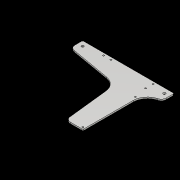
# Autodesk Inventor part: small_gpu_04
Saved by Autodesk Inventor 2018.2 (Build 222227000, 227)
## iProperties
Created: 2020-06-13
Part Number: small_gpu_04
Material: アルミニウム 6061
Document SubType Name: Modeling
Designer: gisen
Density: 2.7 g/cm^3
Appearance: アルミニウム - フラット
Author: gisen
Autodesk Inventor part; units mm, degrees
ref_plane "YZ Plane" through (0, 0, 0) normal (1, 0, 0) x (0, 1, 0)
ref_plane "XZ Plane" through (0, 0, 0) normal (0, 1, 0) x (-1, 0, 0)
ref_plane "XY Plane" through (0, 0, 0) normal (0, 0, 1) x (1, 0, 0)
sketch "スケッチ1" plane through (0, 0, 0) normal (0, 0, 1) x (1, 0, 0)
  line L0 (0, 0) -> (130.16, 0)
  line L1 (130.16, 0) -> (130.16, 159.597)
  line L2 (130.16, 159.597) -> (0, 159.597)
  line L3 (0, 159.597) -> (0, 0)
  dimension "d0" = 130.16
  dimension "d1" = 159.597
  constraints: 8 end point, 2 parallel, 1 horizontal, 1 perpendicular
  measures "d0" distance of L1.end L2.end
  measures "d1" distance between parallel lines of L0 L2
extrude "押し出し1" add sketch "スケッチ1" along normal blind 3
sketch "スケッチ2" plane through (0, 0, 3) normal (0, 0, 1) x (1, 0, 0)
  line L0 (126.16, 3.92) -> (126.16, 113.08) construction
  circle A0 centre (126.16, 3.92) radius 1.6
  circle A1 centre (126.16, 113.08) radius 1.6
  line L1 (130.16, 0) -> (130.16, 159.597) projected
  line L2 (0, 0) -> (130.16, 0) projected
  circle A2 centre (121.531, 154.597) radius 1.6
  line L3 (130.16, 159.597) -> (0, 159.597) projected
  line L4 (121.531, 154.597) -> (121.531, 139.097) construction
  circle A3 centre (121.531, 139.097) radius 1.6
  line L5 (18.398, 154.597) -> (33.898, 154.597) construction
  line L6 (0, 159.597) -> (0, 0) construction
  circle A4 centre (18.398, 154.597) radius 1.6
  circle A5 centre (33.898, 154.597) radius 1.6
  dimension "d4" = 3.2
  dimension "d5" = 4
  dimension "d6" = 3.92
  dimension "d7" = 109.16
  dimension "d10" = 5
  dimension "d11" = 8.629
  dimension "d12" = 15.5
  dimension "d13" = 18.398
  dimension "d14" = 5
  dimension "d15" = 15.5
  constraints: 6 centre point, 6 end point, 5 coincident, 5 equal radius, 2 vertical, 1 horizontal
  measures "d4" diameter of A0
  measures "d5" distance between parallel lines of L1 L0
  measures "d6" distance from line of L2 L0.start
  measures "d7" distance of L0.start L0.end
  measures "d10" distance from line of L4.start L3
  measures "d11" distance from line of L1 L4.start
  measures "d12" distance of L4.start L4.end
  measures "d13" distance from line of L6 L5.start
  measures "d14" distance between parallel lines of L5 L3
  measures "d15" distance of L5.start L5.end
extrude "押し出し2" cut sketch "スケッチ2" against normal blind 3
sketch "スケッチ4" plane through (0, 0, 3) normal (0, 0, 1) x (1, 0, 0)
  line L0 (130.16, 159.597) -> (0, 159.597) construction
  line L1 (130.16, 0) -> (130.16, 159.597) construction
  line L2 (0, 159.597) -> (0, 0) construction
  line L3 (0, 159.597) -> (-30, 159.597)
  line L4 (-30, 159.597) -> (-30, 129.597)
  line L5 (-30, 129.597) -> (0, 129.597)
  line L6 (0, 129.597) -> (0, 159.597)
  line L7 (130.16, 159.597) -> (160.16, 159.597)
  line L8 (160.16, 159.597) -> (160.16, 129.597)
  line L9 (160.16, 129.597) -> (130.16, 129.597)
  line L10 (130.16, 129.597) -> (130.16, 159.597)
  circle A0 centre (-20, 149.597) radius 2.6
  circle A1 centre (150.16, 149.597) radius 2.6
  dimension "d23" = 30
  dimension "d24" = 30
  dimension "d26" = 10
  dimension "d27" = 10
  dimension "d28" = 10
  dimension "d29" = 10
  dimension "d30" = 5.2
  constraints: 16 end point, 4 parallel, 2 centre point, 2 equal length, 2 horizontal, 2 perpendicular, 1 equal radius
  measures "d23" distance of L5.end L4.end
  measures "d24" distance of L4.end L3.end
  measures "d26" distance from line of A0.centre L3
  measures "d27" distance from line of L4 A0.centre
  measures "d28" distance from line of A1.centre L7
  measures "d29" distance from line of L8 A1.centre
  measures "d30" diameter of A0
extrude "押し出し4" add sketch "スケッチ4" against normal blind 3
sketch "スケッチ3" plane through (0, 0, 3) normal (0, 0, 1) x (1, 0, 0)
  circle A0 centre (55.16, 89.597) radius 30 construction
  line L0 (0, 159.597) -> (0, 0) construction
  line L1 (0, 129.597) -> (60.2796, 119.1569)
  line L2 (84.9814, 92.8656) -> (95.16, 0)
  line L3 (0, 0) -> (130.16, 0) construction
  line L4 (130.16, 159.597) -> (0, 159.597) construction
  line L5 (130.16, 0) -> (130.16, 159.597) construction
  arc A1 (84.9814, 92.8656) -> (60.2796, 119.1569) centre (55.16, 89.597) ccw
  line L6 (0, 129.597) -> (0, 0)
  line L7 (0, 0) -> (95.16, 0)
  dimension "d16" = 30
  dimension "d17" = 35
  dimension "d18" = 70
  dimension "d19" = 75
  dimension "d20" = 60
  constraints: 8 end point, 4 point on circle, 3 tangent, 2 centre point, 2 point on line, 1 concentric
  measures "d16" distance of L1.start L0.start
  measures "d17" distance of L3.end L2.end
  measures "d18" distance from line of L4 A0.centre
  measures "d19" distance from line of L5 A0.centre
  measures "d20" diameter of A0
extrude "押し出し3" cut sketch "スケッチ3" against normal blind 3
sketch "スケッチ5" plane through (0, 0, 3) normal (0, 0, 1) x (1, 0, 0)
  line L0 (-30, 159.597) -> (160.16, 159.597) construction
  line L1 (65.08, 159.597) -> (65.08, 0) construction
  line L2 (0, 129.597) -> (60.2796, 119.1569) construction
  line L3 (0, 129.597) -> (-30, 134.7928)
  line L4 (-30, 134.7928) -> (-30, 129.597)
  line L5 (-30, 129.597) -> (0, 129.597)
  line L6 (130.16, 129.597) -> (160.16, 134.7928)
  line L7 (160.16, 134.7928) -> (160.16, 129.597)
  line L8 (160.16, 129.597) -> (130.16, 129.597)
  point P0 (0, 0)
  constraints: 14 end point, 4 symmetric about line, 2 coincident, 2 vertical, 1 collinear, 1 midpoint
extrude "押し出し5" cut sketch "スケッチ5" against normal blind 3
fillet "フィレット1" radius 30 1 edges at (130.16, 129.597, 1.5)
fillet "フィレット2" radius 10 3 edges at (-30, 134.7928, 1.5) (160.16, 134.7928, 1.5) (95.16, 0, 1.5)
fillet "フィレット2" radius 2 3 edges at (130.16, 0, 1.5) (-30, 159.597, 1.5) (160.16, 159.597, 1.5)
equation "\"d28\" = d26"
equation "\"d29\" = d27"
